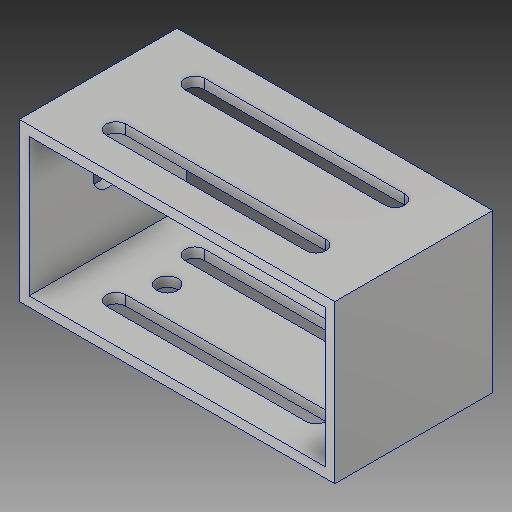
# Autodesk Inventor part: StopMechanismHousing
Saved by Autodesk Inventor 2017 (Build 210142000, 142)
## iProperties
Created: 2016-02-17
Part Number: StopMechanismHousing
Material: Aluminum 6061
Document SubType Name: Modeling
Designer: steele
Density: 2.7 g/cm^3
Appearance: Aluminum - Flat
Mass: 111.493 g
Surface Area: 298.499 cm^2
Volume: 41.2939 cm^3
Author: steele
Autodesk Inventor part; units mm, degrees
ref_plane "YZ Plane" through (0, 0, 0) normal (1, 0, 0) x (0, 1, 0)
ref_plane "XZ Plane" through (0, 0, 0) normal (0, 1, 0) x (-1, 0, 0)
ref_plane "XY Plane" through (0, 0, 0) normal (0, 0, 1) x (1, 0, 0)
sketch "Sketch1" plane through (0, 0, 0) normal (0, 0, 1) x (1, 0, 0)
  line L0 (0, 0) -> (0, 25.4)
  line L1 (0, 25.4) -> (101.6, 25.4)
  line L2 (101.6, 25.4) -> (101.6, 22.225)
  line L3 (98.425, 22.225) -> (3.175, 22.225)
  line L4 (3.175, 22.225) -> (3.175, 0)
  line L5 (0, 0) -> (3.175, 0) construction
  line L6 (0, 0) -> (0, -25.4)
  line L7 (0, -25.4) -> (101.6, -25.4)
  line L8 (101.6, -25.4) -> (101.6, -22.225)
  line L9 (98.425, -22.225) -> (3.175, -22.225)
  line L10 (3.175, -22.225) -> (3.175, 0)
  line L11 (101.6, -25.4) -> (98.425, -25.4)
  line L12 (98.425, -22.225) -> (98.425, 22.225)
  line L13 (98.425, 25.4) -> (101.6, 25.4)
  line L14 (101.6, 25.4) -> (101.6, -25.4)
  dimension "d0" = 25.4
  dimension "d1" = 3.175
  dimension "d2" = 3.175
  dimension "d3" = 101.6
  dimension "d20" = 3.175
  constraints: 30 end point, 4 perpendicular, 4 symmetric about line, 2 horizontal, 2 parallel, 2 vertical, 1 point on line
  measures "d0" distance of L0.start L0.end
  measures "d1" distance between parallel lines of L3 L1
  measures "d2" distance between parallel lines of L4 L0
  measures "d3" distance between parallel lines of L2 L0
  measures "d20" distance between parallel lines of L14 L12
extrude "Extrusion5" add sketch "Sketch1" along normal mid plane 50.8
sketch "Sketch5" plane through (0, 25.4, 25.4) normal (0, 1, 0) x (1, 0, 0)
  line L0 (18.4599, 38.1) -> (82.8223, 38.1) construction
  line L1 (18.4599, 41.275) -> (82.8223, 41.275)
  line L2 (82.8223, 34.925) -> (18.4599, 34.925)
  arc A0 (18.4599, 41.275) -> (18.4599, 34.925) centre (18.4599, 38.1) ccw
  arc A1 (82.8223, 34.925) -> (82.8223, 41.275) centre (82.8223, 38.1) ccw
  line L3 (18.4599, 12.7) -> (82.8223, 12.7) construction
  line L4 (18.4599, 9.525) -> (82.8223, 9.525)
  line L5 (82.8223, 15.875) -> (18.4599, 15.875)
  arc A2 (18.4599, 15.875) -> (18.4599, 9.525) centre (18.4599, 12.7) ccw
  arc A3 (82.8223, 9.525) -> (82.8223, 15.875) centre (82.8223, 12.7) ccw
  line L6 (0, 50.8) -> (101.6, 50.8) projected
  line L7 (101.6, 0) -> (0, 0) projected
  point P0 (0, 25.4)
  point P1 (50.6411, 38.1)
  point P2 (50.6411, 12.7)
  dimension "d23" = 12.7
  dimension "d24" = 12.7
  dimension "d25" = 64.3624
  dimension "d26" = 3.175
  constraints: 16 end point, 8 point on circle, 8 tangent, 4 centre point, 3 parallel, 2 midpoint, 1 equal radius, 1 horizontal
  measures "d23" distance between parallel lines of L0 L6
  measures "d24" distance between parallel lines of L7 L3
  measures "d25" distance of L0.end L0.start
  measures "d26" radius of A0
extrude "Extrusion6" cut sketch "Sketch5" against normal through all
sketch "Sketch6" plane through (0, -25.4, 25.4) normal (-1, 0, 0) x (0, 0, 1)
  circle A0 centre (-25.4, 25.4) radius 4.7625
  dimension "d29" = 9.525
  constraints: 1 centre point, 1 coincident
  measures "d29" diameter of A0
extrude "Extrusion7" cut sketch "Sketch6" against normal up to next
sketch "Sketch8" plane through (3.175, -22.225, -25.4) normal (0, 1, 0) x (1, 0, 0)
  point P0 (19.05, -25.4127)
hole "Hole2" at (22.225, -22.225, 0.0127) direction (0, -1, 0) diameter 6.7564 depth 3.175
sketch "Sketch9" plane through (3.175, -22.225, -25.4) normal (0, 1, 0) x (1, 0, 0)
  point P0 (84.074, -22.1107)
hole "Hole4" at (87.249, -22.225, -3.2893) direction (0, -1, 0) diameter 6.7564 depth 3.175
equation "\"d0\" = 0.5 * stopMechanismLength"
equation "\"d1\" = materialThickness"
equation "\"d2\" = materialThickness"
equation "\"d3\" = stopMEchamismHeight"
equation "\"d20\" = materialThickness"
equation "\"d21\" = stopMechanismWidth"
equation "\"d23\" = slotDistanceFromEdge"
equation "\"d24\" = slotDistanceFromEdge"
equation "\"d26\" = slotRadisu"
equation "\"d27\" = stopMechanismWidth"
equation "\"d29\" = stopMechanismHoleForPost"
equation "\"d30\" = stopMechanismWidth"
equation "\"stopMechanismWidth\" = 50.8"
equation "\"materialThickness\" = 3.175"
equation "\"stopMechanismLength\" = 50.8"
equation "\"stopMEchamismHeight\" = 101.6"
equation "\"stopMechanismHoleForPost\" = 9.525"
equation "\"slotRadisu\" = 0.5 * slotDiam"
equation "\"slotDistanceFromEdge\" = 12.7"
equation "\"slotLengtth\" = 76.2"
equation "\"slotCenterFromFront\" = 50.8"
equation "\"slotDiam\" = 6.35"
body "Solid1"
body "Solid2"
